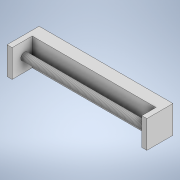
# Autodesk Inventor part: linear trail
Saved by Autodesk Inventor 2022 (Build 260153000, 153)
## iProperties
Created: 2019-07-25
Part Number: linear trail
Material: Generic
Document SubType Name: Modeling
Designer: shenglab2
Density: 1 g/cm^3
Appearance: Default
Author: shenglab2
Autodesk Inventor part; units mm, degrees
ref_plane "YZ Plane" through (0, 0, 0) normal (1, 0, 0) x (0, 1, 0)
ref_plane "XZ Plane" through (0, 0, 0) normal (0, 1, 0) x (-1, 0, 0)
ref_plane "XY Plane" through (0, 0, 0) normal (0, 0, 1) x (1, 0, 0)
sketch "Sketch1" plane through (0, 0, 0) normal (0, 0, 1) x (1, 0, 0)
  line L0 (73, -15) -> (-73, -15)
  line L1 (-73, -15) -> (-73, 15)
  line L2 (-73, 15) -> (73, 15)
  line L3 (73, 15) -> (73, -15)
  line L4 (73, -15) -> (-73, 15) construction
  line L5 (-73, -15) -> (73, 15) construction
  point P0 (0, 0)
  dimension "d0" = 146
  dimension "d1" = 30
  constraints: 12 end point, 2 midpoint, 2 parallel, 1 horizontal, 1 perpendicular
  measures "d0" distance of L1.end L2.end
  measures "d1" distance of L0.end L1.end
extrude "Extrusion1" add sketch "Sketch1" along normal blind 13
sketch "Sketch2" plane through (0, 0, 13) normal (0, 0, 1) x (1, 0, 0)
  line L0 (-73, 15) -> (-73, -15) projected
  line L1 (-73, -15) -> (73, -15) projected
  line L2 (73, -15) -> (73, 15) projected
  line L3 (73, 15) -> (-73, 15) projected
  line L4 (-67.5, 15) -> (-67.5, -15)
  line L5 (67.5, 15) -> (67.5, -15)
  point P0 (0, 0)
  dimension "d4" = 5.5
  dimension "d5" = 5.5
  constraints: 4 end point, 4 point on line, 2 perpendicular
  measures "d4" distance between parallel lines of L0 L4
  measures "d5" distance between parallel lines of L2 L5
extrude "Extrusion2" add sketch "Sketch2" along normal blind 22 contours L3 L4 L1 L0
extrude "Extrusion3" add sketch "Sketch2" along normal blind 15.5 contours L3 L2 L1 L5
sketch "Sketch3" plane through (-67.5, -15, 13) normal (1, 0, 0) x (0, 0, -1)
  line L0 (-22, 0) -> (0, 30)
  circle A0 centre (-11, 15) radius 4.5
  line L1 (-22, 0) -> (-22, 30) projected
  line L2 (-22, 15) -> (-12.5, 15)
  line L3 (-12.5, 15) -> (-8.5, 15)
  circle A1 centre (-8.5, 15) radius 4
  point P0 (13, 15)
  dimension "d10" = 9
  dimension "d21" = 9.5
  dimension "d22" = 4
  constraints: 6 end point, 2 horizontal, 2 midpoint, 1 centre point, 1 coincident, 1 horizontal alignment, 2 other
  measures "d10" diameter of A0
  measures "d21" distance of L2.start L2.end
  measures "d22" distance of L2.end L3.end
extrude "Extrusion7" add sketch "Sketch3" along normal up to surface (135 mm away) contours A1 L3 L0 | L0 A0 A1 | A0 L0 A1 | L3 A1 A0 L0 | A1 L0 A0 picked at (-9.6413, 12.9367) picked at (-5.914, 15.6712) picked at (-8.2588, 18.8681)
thread "Thread2" size "M8x1.25" class "6g" standard "ANSI Metric M Profile" full length
body "Solid1"
